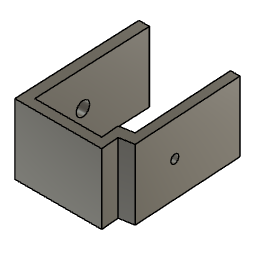
livebox5holder (Autodesk Fusion 360 design; units mm, degrees)
Autodesk Fusion 360 part; units mm, degrees
sketch "Esquisse2" plane through (0, 0, 0) normal (0, 0, 1) x (1, 0, 0)
  line L0 (0, 0) -> (33.5, 0)
  line L1 (0, 0) -> (-2.6172, 59.9429)
  line L2 (0, 0) -> (60, 0) construction
  line L3 (33.5, 0) -> (32.7156, 8.9658)
  line L4 (33.5, 0) -> (42.4658, 0) construction
  line L5 (32.7156, 8.9658) -> (40.0032, 10.2507)
  line L6 (32.7156, 8.9658) -> (40.1156, 8.9658) construction
  line L7 (40.0032, 10.2507) -> (36.8897, 61.1556)
  line L8 (40.0032, 10.2507) -> (91.0032, 10.2507) construction
  line L9 (36.8897, 61.1556) -> (-2.6172, 59.9429)
  dimension "d13" = 33.5
  dimension "d14" = 92.5
  dimension "d15" = 60
  dimension "d16" = 95
  dimension "d17" = 9
  dimension "d18" = 10
  dimension "d19" = 7.4
  dimension "d20" = 93.5
  dimension "d21" = 51
  constraint coincident L0.start L1.start
  constraint horizontal L0
  constraint horizontal L2
  constraint horizontal L4
  constraint horizontal L6
  constraint horizontal L8
  measures "d13" distance of L0.start L0.end
  measures "d14" angle of L1 L2
  measures "d15" distance of L0.start L1.end
  measures "d16" angle of L3 L4
  measures "d17" distance of L0.end L3.end
  measures "d18" angle of L5 L6
  measures "d19" distance of L3.end L5.end
  measures "d20" angle of L7 L8
  measures "d21" distance of L5.end L7.end
sketch "Esquisse3" plane through (0, 0, 0) normal (0, 0, 1) x (1, 0, 0)
  line L0 (0, 0) -> (-5, 0) construction
  line L1 (-5, 0) -> (-5, -5) construction
  line L2 (-5, -5) -> (0, -5) construction
  line L3 (0, -5) -> (0, 0) construction
  line L4 (-5, -5) -> (38.5, -5)
  line L5 (-5, -5) -> (-7.8353, 59.9381)
  line L6 (-5, -5) -> (65, -5) construction
  line L7 (38.5, -5) -> (37.7156, 3.9658)
  line L8 (38.5, -5) -> (47.4658, -5) construction
  line L9 (37.7156, 3.9658) -> (45.0032, 5.2507)
  line L10 (37.7156, 3.9658) -> (45.1156, 3.9658) construction
  line L11 (45.0032, 5.2507) -> (41.5845, 61.1463)
  line L12 (45.0032, 5.2507) -> (106.0032, 5.2507) construction
  line L13 (-7.8353, 59.9381) -> (41.5845, 61.1463)
  dimension "d22" = 5
  dimension "d23" = 5
  dimension "d24" = 43.5
  dimension "d25" = 92.5
  dimension "d26" = 65
  dimension "d27" = 95
  dimension "d28" = 9
  dimension "d29" = 10
  dimension "d30" = 7.4
  dimension "d31" = 93.5
  dimension "d32" = 56
  constraint horizontal L0
  constraint vertical L1
  constraint horizontal L2
  constraint vertical L3
  constraint coincident L0.start L3.end
  constraint perpendicular L1 L4
  constraint horizontal L6
  constraint horizontal L8
  constraint horizontal L10
  constraint horizontal L12
  measures "d22" distance of L0.start L0.end
  measures "d23" distance of L0.start L2.end
  measures "d24" distance of L1.end L4.end
  measures "d25" angle of L5 L6
  measures "d26" distance of L1.end L5.end
  measures "d27" angle of L7 L8
  measures "d28" distance of L4.end L7.end
  measures "d29" angle of L9 L10
  measures "d30" distance of L7.end L9.end
  measures "d31" angle of L11 L12
  measures "d32" distance of L9.end L11.end
extrude "Extrusion1" add sketch "Esquisse3" along normal blind 35
extrude "Extrusion2" cut sketch "Esquisse2" along normal blind 35
extrude "Extrusion3" cut 1 faces at (10.4829, 60.345, 23.3333) along direction (-0.030682, 0.999529, 0) blind 10
ref_plane "Plan de construction1" through (36.8973, 61.0317, 35) normal (-0.998135, -0.061049, 0) x (0.061049, -0.998135, 0)
sketch "Esquisse4" plane through (36.8973, 61.0317, 35) normal (-0.998135, -0.061049, 0) x (0.061049, -0.998135, 0)
  line L0 (0, 0) -> (35, 0) construction
  line L1 (35, 0) -> (35, -17.5) construction
  line L2 (35, -17.5) -> (0, -17.5) construction
  line L3 (0, -17.5) -> (0, 0) construction
  circle A0 centre (35, -17.5) radius 3.8
  dimension "d41" = 35
  dimension "d42" = 17.5
  dimension "d43" = 7.6
  constraint horizontal L0
  constraint vertical L1
  constraint horizontal L2
  constraint vertical L3
  constraint coincident L0.start L3.end
  constraint coincident L1.end L2.start
  measures "d41" distance of L0.start L0.end
  measures "d42" distance of L0.start L2.end
  measures "d43" diameter of A0
ref_plane "Plan de construction2" through (44.0247, 26.4022, 17.5) normal (-0.998135, -0.061049, 0) x (0.061049, -0.998135, 0)
sketch "Esquisse5" plane through (44.0247, 26.4022, 17.5) normal (-0.998135, -0.061049, 0) x (0.061049, -0.998135, 0)
  circle A0 centre (0, 0) radius 2
  dimension "d45" = 4
  constraint coincident A0.centre origin
  measures "d45" diameter of A0
loft "Lissage1" cut profiles "Esquisse5", "Esquisse4" section 1 section 2
ref_plane "Plan de construction3" through (-7.8353, 59.9381, 35) normal (-0.999048, -0.043619, 0) x (0.043619, -0.999048, 0)
sketch "Esquisse6" plane through (-7.8353, 59.9381, 35) normal (-0.999048, -0.043619, 0) x (0.043619, -0.999048, 0)
  line L0 (0, 0) -> (35, 0) construction
  line L1 (35, 0) -> (35, -17.5) construction
  line L2 (35, -17.5) -> (0, -17.5) construction
  line L3 (0, -17.5) -> (0, 0) construction
  circle A0 centre (35, -17.5) radius 3.5
  dimension "d46" = 35
  dimension "d47" = 17.5
  dimension "d48" = 7
  constraint horizontal L0
  constraint vertical L1
  constraint horizontal L2
  constraint vertical L3
  constraint coincident L0.start L3.end
  constraint coincident L1.end L2.start
  measures "d46" distance of L0.start L0.end
  measures "d47" distance of L0.start L2.end
  measures "d48" diameter of A0
extrude "Extrusion4" cut sketch "Esquisse6" against normal blind 10
equation "height = 60 mm"
equation "bottomWidth = 33.5 mm"
equation "edgeHeight = 9 mm"
equation "edgeWidth = 7.4 mm"
equation "thickness = 5 mm"
equation "screwHoleDiameter = 4 mm"
equation "screwHoleBevel = 7.6 mm"
equation "screwDriverHoleDiameter = 7 mm"
equation "angle1 = 92.5 deg"
equation "angle2 = 95 deg"
equation "angle3 = 10 deg"
equation "angle4 = 93.5 deg"
equation "d13 = bottomWidth"
equation "d14 = angle1"
equation "d15 = height"
equation "d16 = angle2"
equation "d18 = angle3"
equation "d19 = edgeWidth"
equation "d20 = angle4"
equation "d21 = height - edgeHeight"
equation "d22 = thickness"
equation "d23 = thickness"
equation "d24 = bottomWidth + ( 2 * thickness )"
equation "d25 = angle1"
equation "d26 = height + thickness"
equation "d27 = angle2"
equation "d28 = edgeHeight"
equation "d29 = angle3"
equation "d30 = edgeWidth"
equation "d31 = angle4"
equation "d32 = height - edgeHeight + thickness"
equation "d33 = width"
equation "width = 35 mm"
equation "d36 = width"
equation "screwHoleHeight = 30 mm"
equation "d41 = height + thickness - screwHoleHeight"
equation "d42 = width / 2"
equation "d43 = screwHoleBevel"
equation "d44 = -thickness"
equation "d45 = screwHoleDiameter"
equation "d46 = height + thickness - screwHoleHeight"
equation "d47 = width / 2"
equation "d48 = screwDriverHoleDiameter"
equation "d49 = -thickness * 2"
